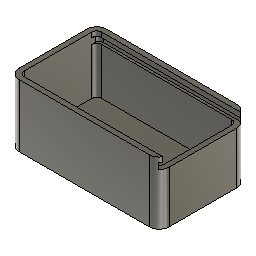
boite_domino v26 (Autodesk Fusion 360 design; units mm, degrees)
Autodesk Fusion 360 part; units mm, degrees
sketch "Esquisse1" plane through (0, 0, 0) normal (0, 0, 1) x (1, 0, 0) in component "boite"
  line L0 (26, 17.5) -> (-26, 17.5)
  line L1 (-30, 13.5) -> (-30, -13.5)
  line L2 (-26, -17.5) -> (26, -17.5)
  line L3 (30, -13.5) -> (30, 13.5)
  line L4 (30, 17.5) -> (-30, -17.5) construction
  line L5 (-30, 17.5) -> (30, -17.5) construction
  arc A0 (-26, 17.5) -> (-30, 13.5) centre (-26, 13.5) ccw
  arc A1 (-30, -13.5) -> (-26, -17.5) centre (-26, -13.5) ccw
  arc A2 (30, 13.5) -> (26, 17.5) centre (26, 13.5) ccw
  arc A3 (26, -17.5) -> (30, -13.5) centre (26, -13.5) ccw
  dimension "d8" = 60
  dimension "d9" = 35
  dimension "d10" = 4
  constraint horizontal L0
  constraint perpendicular L0 L1
  constraint parallel L0 L2
  constraint parallel L1 L3
  constraint coincident L4 origin
  constraint coincident L5 origin
  constraint coincident L5.start L1
  constraint coincident L5.start L0
  constraint tangent L1 A0
  constraint tangent L0 A0
  constraint coincident L4.end L1
  constraint coincident L4.end L2
  constraint tangent L1 A1
  constraint tangent L2 A1
  constraint equal A0 A1
  constraint coincident L4.start L0
  constraint coincident L4.start L3
  constraint tangent L0 A2
  constraint tangent L3 A2
  constraint equal A0 A2
  constraint coincident L5.end L3
  constraint coincident L5.end L2
  constraint tangent L3 A3
  constraint tangent L2 A3
  constraint equal A0 A3
  measures "d8" distance of L4.end L5.end
  measures "d9" distance of L5.start L4.end
  measures "d10" radius of A0
extrude "Extrusion1" add sketch "Esquisse1" along normal blind 25 makes body 1 in component "boite"
sketch "Esquisse2" plane through (0, 0, 25) normal (0, 0, 1) x (-1, 0, 0) in component "boite"
  arc A0 (-26, 17.5) -> (-30, 13.5) centre (-26, 13.5) ccw
  line L0 (-30, 13.5) -> (-30, -13.5)
  arc A1 (-30, -13.5) -> (-26, -17.5) centre (-26, -13.5) ccw
  line L1 (-26, -17.5) -> (26, -17.5)
  arc A2 (26, -17.5) -> (30, -13.5) centre (26, -13.5) ccw
  line L2 (30, -13.5) -> (30, 13.5)
  arc A3 (30, 13.5) -> (26, 17.5) centre (26, 13.5) ccw
  line L3 (26, 17.5) -> (-26, 17.5)
  line L4 (-28, 13.5) -> (-28, -13.5)
  arc A4 (-28, -13.5) -> (-26, -15.5) centre (-26, -13.5) ccw
  line L5 (-26, -15.5) -> (26, -15.5)
  arc A5 (26, -15.5) -> (28, -13.5) centre (26, -13.5) ccw
  line L6 (28, -13.5) -> (28, 13.5)
  arc A6 (28, 13.5) -> (26, 15.5) centre (26, 13.5) ccw
  line L7 (26, 15.5) -> (-26, 15.5)
  arc A7 (-26, 15.5) -> (-28, 13.5) centre (-26, 13.5) ccw
extrude "Extrusion2" cut sketch "Esquisse2" against normal blind 23 contours L4 A4 L5 A5 L6 A6 L7 A7 bodies 1 in component "boite"
sketch "Esquisse3" plane through (30, 0, 0) normal (1, 0, 0) x (0, 1, 0) in component "boite"
  line L0 (-13.5, 0) -> (13.5, 0)
  line L1 (13.5, 0) -> (13.5, 25)
  line L2 (13.5, 25) -> (-13.5, 25)
  line L3 (-13.5, 25) -> (-13.5, 0)
  line L4 (-16.5, 23) -> (16.5, 23)
  line L5 (16.5, 23) -> (16.5, 20.7)
  line L6 (16.5, 20.7) -> (-16.5, 20.7)
  line L7 (-16.5, 20.7) -> (-16.5, 23)
  line L8 (-16.5, 23) -> (16.5, 20.7) construction
  line L9 (16.5, 23) -> (-16.5, 20.7) construction
  line L10 (-17.5, 0) -> (-17.5, 25)
  line L11 (-15.5, 23) -> (15.5, 23)
  line L12 (15.5, 23) -> (15.5, 25)
  line L13 (15.5, 25) -> (-15.5, 25)
  line L14 (-15.5, 25) -> (-15.5, 23)
  line L15 (-15.5, 23) -> (15.5, 25) construction
  line L16 (15.5, 23) -> (-15.5, 25) construction
  line L17 (-13.5, 25) -> (13.5, 25)
  line L18 (17.5, 0) -> (17.5, 25)
  point P0 (0, 21.85)
  point P1 (0, 24)
  dimension "d16" = 33
  dimension "d17" = 2.3
  dimension "d18" = 2
  dimension "d68" = 17.5
  dimension "d136" = 2
  dimension "d137" = 2
  dimension "d138" = 2
  constraint horizontal L4
  constraint perpendicular L4 L5
  constraint parallel L4 L6
  constraint parallel L5 L7
  constraint coincident L8 P0
  constraint coincident L9 P0
  constraint horizontal L11
  constraint perpendicular L11 L12
  constraint parallel L11 L13
  constraint parallel L12 L14
  constraint coincident L15 P1
  constraint coincident L16 P1
  constraint coincident L13 L2.end
  measures "d16" distance of L4.start L4.end
  measures "d17" distance of L4.start L6.end
  measures "d18" distance of L2 L4
  measures "d68" distance of P0 L10
  measures "d136" distance of L10 L14
  measures "d137" distance of L12 L18
  measures "d138" distance of L11 L13
extrude "Extrusion3" cut sketch "Esquisse3" against normal blind 58 contours L3 L4 L6 L7 L11 | L1 L3 L4 L6 L11 | L1 L4 L5 L6 L11 | L3 L4 L11 L13 L14 | L1 L2 L3 L4 L11 L13 L17 | L1 L4 L11 L12 L13 bodies 1 in component "boite"
fillet "Congé15" radius 2 2 edges at (-28, -15.5, 24) (-28, 15.5, 24) on bodies 1 in component "boite"
fillet "Congé16" radius 1.7 2 edges at (-28, -16.5, 21.85) (-28, 16.5, 21.85) on bodies 1 in component "boite"
sketch "Esquisse1 (2)" plane through (30, 0, 0) normal (1, 0, 0) x (0, 1, 0) in component "couvercle"
  line L0 (13.5, 20.7) -> (-13.5, 20.7)
  line L1 (-13.5, 20.7) -> (-13.5, 0)
  line L2 (-13.5, 0) -> (13.5, 0)
  line L3 (13.5, 0) -> (13.5, 20.7)
  line L4 (-16.2, 22.7) -> (16.2, 22.7)
  line L5 (16.2, 22.7) -> (16.2, 21)
  line L6 (16.2, 21) -> (-16.2, 21)
  line L7 (-16.2, 21) -> (-16.2, 22.7)
  line L8 (-16.2, 22.7) -> (16.2, 21) construction
  line L9 (16.2, 22.7) -> (-16.2, 21) construction
  line L10 (-16.5, 20.7) -> (-16.5, 23)
  line L11 (16.5, 23) -> (16.5, 20.7)
  line L12 (-15.5, 23) -> (-16.5, 23)
  line L13 (-16.5, 20.7) -> (-13.5, 20.7)
  line L14 (-30.7, 25) -> (30.7, 25)
  line L15 (30.7, 25) -> (30.7, 21.5889)
  line L16 (30.7, 21.5889) -> (-30.7, 21.5889)
  line L17 (-30.7, 21.5889) -> (-30.7, 25)
  line L18 (-30.7, 25) -> (30.7, 21.5889) construction
  line L19 (30.7, 25) -> (-30.7, 21.5889) construction
  line L20 (-31, 48) -> (-31, 50)
  line L21 (31, 48) -> (31, 50)
  line L22 (-13.5, 25) -> (13.5, 25)
  point P0 (0, 21.85)
  point P1 (0, 23.2944)
  dimension "d109" = 0.3
  dimension "d110" = 0.3
  dimension "d112" = 0.3
  dimension "d114" = 0.3
  dimension "d115" = 0.3
  dimension "d116" = 0.3
  constraint horizontal L4
  constraint perpendicular L4 L5
  constraint parallel L4 L6
  constraint parallel L5 L7
  constraint coincident L8 P0
  constraint coincident L9 P0
  constraint horizontal L14
  constraint perpendicular L14 L15
  constraint parallel L14 L16
  constraint parallel L15 L17
  constraint coincident L18 P1
  constraint coincident L19 P1
  constraint coincident L14.start L22
  measures "d109" distance of L7 L10
  measures "d110" distance of L5 L11
  measures "d112" distance of L4 L12
  measures "d114" distance of L6 L13
  measures "d115" distance of L17 L20
  measures "d116" distance of L15 L21
extrude "Extrusion1'" add sketch "Esquisse1 (2)" against normal up to surface (58 mm away) separate body contours L4 L5 L7 L16 | L5 L6 L7 L16 makes body 2 in component "couvercle"
fillet "Congé1" radius 1.7 2 edges at (-28, -16.2, 21.85) (-28, 16.2, 21.85) on bodies 2 in component "couvercle"
sketch "Esquisse5" plane through (0, 0, 22.7) normal (0, 0, 1) x (-1, 0, 0) in component "couvercle"
  arc A0 (26.3, -16.2) -> (28, -14.5) centre (26.3, -14.5) ccw
  line L0 (28, -14.5) -> (28, 14.5)
  arc A1 (28, 14.5) -> (26.3, 16.2) centre (26.3, 14.5) ccw
  line L1 (26.3, 16.2) -> (-30, 16.2)
  line L2 (-30, 16.2) -> (-30, -16.2)
  line L3 (-30, -16.2) -> (26.3, -16.2)
  arc A2 (-26, 17.5) -> (-29.4641, 15.5) centre (-26, 13.5) ccw
  line L4 (-30, 16.2) -> (26.3, 16.2)
  line L5 (-30, 16.2) -> (-30, -16.2)
  line L6 (-30, -16.2) -> (26.3, -16.2)
  arc A3 (-29.4641, -15.5) -> (-26, -17.5) centre (-26, -13.5) ccw
  arc A4 (-30, -13.5) -> (-26, -17.5) centre (-26, -13.5) ccw
  arc A5 (-26, 17.5) -> (-30, 13.5) centre (-26, 13.5) ccw
sketch "Esquisse9" plane through (0, 0, 22.7) normal (0, 0, 1) x (-1, 0, 0)
  arc A0 (26.3, -16.2) -> (28, -14.5) centre (26.3, -14.5) ccw
  line L0 (28, -14.5) -> (28, 14.5)
  arc A1 (28, 14.5) -> (26.3, 16.2) centre (26.3, 14.5) ccw
  line L1 (26.3, 16.2) -> (-30, 16.2)
  line L2 (-30, 16.2) -> (-30, -16.2)
  line L3 (-30, -16.2) -> (26.3, -16.2)
  arc A2 (-30, -13.5) -> (-28.6458, -16.5) centre (-26, -13.5) ccw
  arc A3 (-28.6458, 16.5) -> (-30, 13.5) centre (-26, 13.5) ccw
extrude "Extrusion6" cut sketch "Esquisse9" against normal blind 2 contours L2 L3 A2 | L1 L2 A3 bodies 2 in component "couvercle"
sketch "Esquisse10" plane through (0, 0, 22.7) normal (0, 0, 1) x (-1, 0, 0)
  arc A0 (-30, -13.5) -> (-28.9513, -16.2) centre (-26, -13.5) ccw
  line L0 (-28.9513, -16.2) -> (26.3, -16.2)
  arc A1 (26.3, -16.2) -> (28, -14.5) centre (26.3, -14.5) ccw
  line L1 (28, -14.5) -> (28, 14.5)
  arc A2 (28, 14.5) -> (26.3, 16.2) centre (26.3, 14.5) ccw
  line L2 (26.3, 16.2) -> (-28.9513, 16.2)
  arc A3 (-28.9513, 16.2) -> (-30, 13.5) centre (-26, 13.5) ccw
  line L3 (-30, 13.5) -> (-30, -13.5)
  line L4 (-28, -15.2) -> (-30, -15.2)
  line L5 (-30, -15.2) -> (-30, 15.2)
  line L6 (-30, 15.2) -> (-28, 15.2)
  line L7 (-28, 15.2) -> (-28, -15.2)
  line L8 (-28, -15.2) -> (-30, 15.2) construction
  line L9 (-30, -15.2) -> (-28, 15.2) construction
  line L10 (-30, 13.5) -> (-30, -13.5)
  line L11 (26, -15.5) -> (-29.4641, -15.5)
  line L12 (-29.4641, 15.5) -> (26, 15.5)
  arc A4 (-30, -13.5) -> (-28.9513, -16.2) centre (-26, -13.5) ccw
  arc A5 (-28.9513, 16.2) -> (-30, 13.5) centre (-26, 13.5) ccw
  point P0 (-29, 0)
  dimension "d145" = 2
  dimension "d146" = 0.3
  dimension "d147" = 0.3
  constraint horizontal L4
  constraint perpendicular L4 L5
  constraint parallel L4 L6
  constraint parallel L5 L7
  constraint coincident L8 P0
  constraint coincident L9 P0
  constraint coincident A0.start L5
  measures "d145" distance of L5 L7
  measures "d146" distance of L4 L11
  measures "d147" distance of L6 L12
extrude "Extrusion7" add sketch "Esquisse10" along normal blind 2.3 contours A0 A3 L3 L4 L5 L6 L7 L10 A4 A5 bodies 2 in component "couvercle"
move_body "Déplacer2" bodies 2 to x (1, 0, 0) y (0, 1, 0) z (0, 0, 1) at (30, 0, 0) in component "couvercle"
component "boite" placed x (1, 0, 0) y (0, 1, 0) z (0, 0, 1) at (0, 0, 0)
component "couvercle" placed x (1, 0, 0) y (0, 1, 0) z (0, 0, 1) at (0, 0, 0)
equation "longueur = 60 mm"
equation "largeur = 35 mm"
equation "hauteur = 25 mm"
equation "epaisseur = 2 mm"
equation "rayonext = 4 mm"
equation "rayonint = rayonext - epaisseur"
equation "jeu = 0.3 mm"
equation "d8 = longueur"
equation "d9 = largeur"
equation "d10 = rayonext"
equation "d11 = hauteur"
equation "d13 = -epaisseur"
equation "d14 = -hauteur + epaisseur"
equation "d16 = largeur - epaisseur"
equation "d17 = jeu + epaisseur"
equation "d18 = epaisseur"
equation "d21 = -longueur + epaisseur"
equation "d68 = largeur / 2"
equation "d109 = jeu"
equation "d110 = jeu"
equation "d112 = jeu"
equation "d114 = jeu"
equation "d115 = jeu"
equation "d116 = jeu"
equation "d120 = rayonint - jeu"
equation "d136 = epaisseur"
equation "d137 = epaisseur"
equation "d138 = d18"
equation "d140 = rayonint"
equation "d142 = rayonint - jeu"
equation "d143 = -epaisseur"
equation "d146 = jeu"
equation "d147 = jeu"
equation "d148 = epaisseur + jeu"
